Base v15 (Autodesk Fusion 360 design; units mm, degrees)
Autodesk Fusion 360 part; units mm, degrees
sketch "Sketch1" plane through (0, 0, 0) normal (0, 1, 0) x (1, 0, 0)
  line L0 (0, 0) -> (85, 0)
  line L1 (85, 0) -> (85, -65)
  line L2 (85, -65) -> (0, -65)
  line L3 (0, -65) -> (0, 0)
  dimension "d1" = 65
  dimension "d2" = 85
  constraint horizontal L0
  constraint vertical L1
  constraint horizontal L2
  constraint vertical L3
  constraint coincident L0.start L3.end
extrude "Extrude1" add sketch "Sketch1" along normal blind 10
sketch "Sketch2" plane through (0, 10, 0) normal (0, 1, 0) x (-1, 0, 0)
  line L0 (0, 65) -> (-85, 65)
  line L1 (-85, 65) -> (-85, 0)
  line L2 (-85, 0) -> (0, 0)
  line L3 (0, 0) -> (0, 65)
  line L4 (-3, 0.7) -> (-40.6, 0.7)
  line L5 (-40.6, 0.7) -> (-40.6, 64.3)
  line L6 (-40.6, 64.3) -> (-3, 64.3)
  line L7 (-3, 64.3) -> (-3, 0.7)
  line L8 (0, 32.5) -> (-85, 32.5) construction
  line L9 (-40.6, 32.5) -> (-3, 32.5) construction
  dimension "d5" = 63.6
  dimension "d6" = 37.6
  dimension "d7" = 3
  constraint horizontal L4
  constraint vertical L5
  constraint horizontal L6
  constraint vertical L7
  constraint midpoint L3 L2.end
  constraint midpoint L1 L2.end
  constraint midpoint L5 L2.end
  constraint midpoint L7 L2.end
  constraint collinear L8 L9
  measures "d5" distance of L2.end
  measures "d7" distance of L3 L7
extrude "Extrude2" cut sketch "Sketch2" against normal blind 5 contours L4 L5 L6 L7
sketch "Sketch3" plane through (0, 10, 0) normal (0, 1, 0) x (-1, 0, 0)
  line L0 (-40.6, 0.7) -> (-40.6, 64.3)
  line L1 (-3, 64.3) -> (-3, 0.7)
  line L2 (-3, 0.7) -> (-40.6, 0.7)
  line L3 (0, 65) -> (-85, 65)
  line L4 (-85, 65) -> (-85, 0)
  line L5 (-85, 0) -> (0, 0)
  line L6 (0, 0) -> (0, 65)
  line L7 (-45.6, 1.45) -> (-47.6, 1.45)
  line L8 (-47.6, 1.45) -> (-47.6, 63.55)
  line L9 (-47.6, 63.55) -> (-45.6, 63.55)
  line L10 (-45.6, 63.55) -> (-45.6, 1.45)
  line L11 (-40.6, 64.3) -> (-3, 64.3)
  line L12 (-45.6, 32.5) -> (-47.6, 32.5) construction
  line L13 (0, 32.5) -> (-85, 32.5) construction
  dimension "d12" = 62.1
  dimension "d13" = 2
  dimension "d14" = 5
  constraint horizontal L7
  constraint vertical L8
  constraint horizontal L9
  constraint vertical L10
  constraint midpoint L10 L5.end
  constraint midpoint L8 L5.end
  constraint midpoint L6 L5.end
  constraint midpoint L4 L5.end
  constraint collinear L12 L13
  measures "d14" distance of L0 L10
extrude "Extrude3" cut sketch "Sketch3" against normal blind 7.5 contours L7 L8 L9 L10
sketch "Sketch4" plane through (0, 10, 0) normal (0, 1, 0) x (-1, 0, 0)
  line L0 (-47.6, 1.45) -> (-47.6, 63.55)
  line L1 (-45.6, 63.55) -> (-45.6, 1.45)
  line L2 (-45.6, 1.45) -> (-47.6, 1.45)
  line L3 (-40.6, 0.7) -> (-40.6, 64.3)
  line L4 (-3, 64.3) -> (-3, 0.7)
  line L5 (-3, 0.7) -> (-40.6, 0.7)
  line L6 (0, 65) -> (-85, 65)
  line L7 (-85, 65) -> (-85, 0)
  line L8 (-85, 0) -> (0, 0)
  line L9 (0, 0) -> (0, 65)
  line L10 (-62.6, 1.45) -> (-65.7, 1.45)
  line L11 (-65.7, 1.45) -> (-65.7, 63.55)
  line L12 (-65.7, 63.55) -> (-62.6, 63.55)
  line L13 (-62.6, 63.55) -> (-62.6, 1.45)
  line L14 (-40.6, 64.3) -> (-3, 64.3)
  line L15 (-47.6, 63.55) -> (-45.6, 63.55)
  line L16 (-62.6, 32.5) -> (-65.7, 32.5) construction
  line L17 (-85, 32.5) -> (0, 32.5) construction
  dimension "d17" = 3.1
  dimension "d18" = 15
  dimension "d26" = 62.1
  constraint horizontal L10
  constraint vertical L11
  constraint horizontal L12
  constraint vertical L13
  constraint midpoint L13 L8.end
  constraint midpoint L11 L8.end
  constraint midpoint L7 L8.end
  constraint midpoint L9 L8.end
  constraint collinear L16 L17
  measures "d18" distance of L0 L13
extrude "Extrude4" cut sketch "Sketch4" against normal blind 7.5 contours L10 L11 L12 L13
sketch "Sketch5" plane through (0, 10, 0) normal (0, 1, 0) x (-1, 0, 0)
  line L0 (-65.7, 1.45) -> (-65.7, 63.55)
  line L1 (-62.6, 63.55) -> (-62.6, 1.45)
  line L2 (-62.6, 1.45) -> (-65.7, 1.45)
  line L3 (-47.6, 1.45) -> (-47.6, 63.55)
  line L4 (-45.6, 63.55) -> (-45.6, 1.45)
  line L5 (-45.6, 1.45) -> (-47.6, 1.45)
  line L6 (-40.6, 0.7) -> (-40.6, 64.3)
  line L7 (-3, 64.3) -> (-3, 0.7)
  line L8 (-3, 0.7) -> (-40.6, 0.7)
  line L9 (0, 65) -> (-85, 65)
  line L10 (-85, 65) -> (-85, 0)
  line L11 (-85, 0) -> (0, 0)
  line L12 (0, 0) -> (0, 65)
  line L13 (-80.85, 1.45) -> (-83.95, 1.45)
  line L14 (-83.95, 1.45) -> (-83.95, 63.55)
  line L15 (-83.95, 63.55) -> (-80.85, 63.55)
  line L16 (-80.85, 63.55) -> (-80.85, 1.45)
  line L17 (-40.6, 64.3) -> (-3, 64.3)
  line L18 (-47.6, 63.55) -> (-45.6, 63.55)
  line L19 (-65.7, 63.55) -> (-62.6, 63.55)
  line L20 (-80.85, 32.5) -> (-83.95, 32.5) construction
  line L21 (-85, 32.5) -> (0, 32.5) construction
  dimension "d21" = 3.1
  dimension "d22" = 15.15
  dimension "d27" = 62.1
  constraint horizontal L13
  constraint vertical L14
  constraint horizontal L15
  constraint vertical L16
  constraint midpoint L16 L11.end
  constraint midpoint L14 L11.end
  constraint midpoint L10 L11.end
  constraint midpoint L12 L11.end
  constraint collinear L20 L21
  measures "d22" distance of L0 L16
  measures "d27" distance of L11.end
extrude "Extrude5" cut sketch "Sketch5" against normal blind 7.5 contours L13 L14 L15 L16
fillet "Fillet1" radius 2 4 edges at (85, 5, 65) (85, 5, 0) (0, 5, 0) (0, 5, 65)
